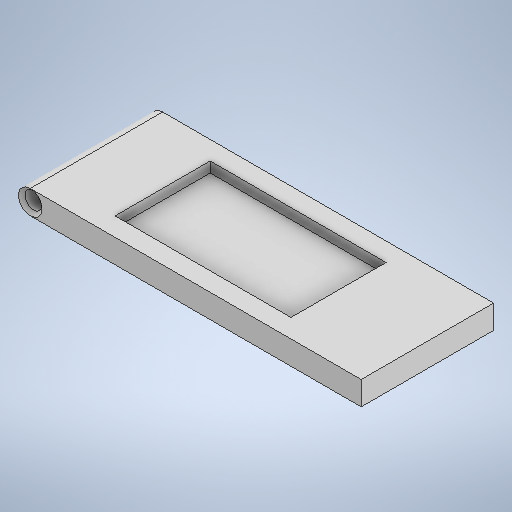
# Autodesk Inventor part: Leaf
Saved by Autodesk Inventor 2025 (Build 290162000, 162)
## iProperties
Created: 2024-06-14
Part Number: Leaf
Material: Generic
Document SubType Name: Modeling
Designer: track
Density: 1 g/cm^3
Appearance: Default
Author: track
Autodesk Inventor part; units mm, degrees
ref_plane "YZ Plane" through (0, 0, 0) normal (1, 0, 0) x (0, 1, 0)
ref_plane "XZ Plane" through (0, 0, 0) normal (0, 1, 0) x (-1, 0, 0)
ref_plane "XY Plane" through (0, 0, 0) normal (0, 0, 1) x (1, 0, 0)
sketch "Sketch2" plane through (0, 0, 0) normal (0, 0, 1) x (1, 0, 0)
  arc A0 (0, 4.545) -> (0, -4.545) centre (0, 0) ccw
  circle A1 centre (0, 0) radius 3.275
  line L0 (0, 4.545) -> (127, 4.545)
  line L1 (0, -4.545) -> (127, -4.545)
  line L2 (127, -4.545) -> (127, 4.545)
  dimension "d0" = 1.27
  dimension "d1" = 6.55
  dimension "d2" = 127
  constraints: 6 end point, 2 centre point, 2 coincident, 2 horizontal, 2 point on circle, 2 tangent, 1 perpendicular
  measures "d0" radial gap between concentric circles of A0 A1
  measures "d1" diameter of A1
  measures "d2" distance of L0.start L0.end
extrude "Extrusion1" add sketch "Sketch2" along normal mid plane 50.8
chamfer "Chamfer1" distance 1.27 angle 45 1 edges at (-3.275, 0, 25.4)
chamfer "Chamfer2" distance 1.27 angle 45 1 edges at (-3.275, 0, -25.4)
sketch "Sketch3" plane through (127, 4.545, 25.4) normal (0, 1, 0) x (1, 0, 0)
  line L0 (-101.6, 7.15) -> (-34.1, 7.15)
  line L1 (-34.1, 7.15) -> (-34.1, 43.65)
  line L2 (-34.1, 43.65) -> (-101.6, 43.65)
  line L3 (-101.6, 43.65) -> (-101.6, 7.15)
  line L4 (0, 0) -> (-127, 0) projected
  line L5 (-127, 50.8) -> (-127, 0) projected
  line L6 (-127, 50.8) -> (0, 50.8) projected
  point P0 (-127, 25.4)
  point P1 (-101.6, 25.4)
  dimension "d12" = 36.5
  dimension "d13" = 67.5
  dimension "d15" = 25.4
  dimension "d16" = 25.4
  constraints: 8 end point, 2 parallel, 1 horizontal, 1 midpoint, 1 perpendicular
  measures "d12" distance of L2.end L0.start
  measures "d13" distance of L1.end L2.end
  measures "d15" distance between parallel lines of L5 L3
  measures "d16" distance from line of L6 point (-101.6, 25.4)
extrude "Extrusion2" cut sketch "Sketch3" against normal blind 4
sketch "Sketch4" plane through (127, -4.545, -25.4) normal (0, -1, 0) x (1, 0, 0)
  line L0 (-119.38, 3.81) -> (-3.81, 3.81)
  line L1 (-3.81, 3.81) -> (-3.81, 46.99)
  line L2 (-3.81, 46.99) -> (-119.38, 46.99)
  line L3 (-119.38, 46.99) -> (-119.38, 3.81)
  line L4 (0, 0) -> (0, 50.8) projected
  line L5 (0, 0) -> (-127, 0) projected
  line L6 (-127, 50.8) -> (0, 50.8) projected
  line L7 (-127, 50.8) -> (-127, 0) projected
  point P0 (-127, 25.4)
  point P1 (-3.81, 25.4)
  dimension "d19" = 3.81
  dimension "d20" = 3.81
  dimension "d21" = 3.81
  dimension "d22" = 7.62
  constraints: 8 end point, 2 parallel, 1 horizontal, 1 midpoint, 1 perpendicular
  measures "d19" distance from line of L4 point (-3.81, 25.4)
  measures "d20" distance between parallel lines of L5 L0
  measures "d21" distance between parallel lines of L6 L2
  measures "d22" distance between parallel lines of L7 L3
extrude "Extrusion3" cut sketch "Sketch4" against normal blind 4 contours L3 L2 L1 L0
body "Solid1"
